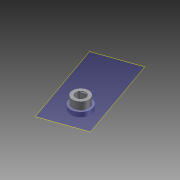
# Autodesk Inventor part: BlankLargeGearMotorInput
Saved by Autodesk Inventor 2012 (Build 160160000, 160)
## iProperties
Created: 2011-10-22
Part Number: BlankLargeGearMotorInput
Material: Default
Document SubType Name: Modeling
Designer: KuttaA
Density: 1 g/cm^3
Mass: 1.83252 g
Surface Area: 19.0134 cm^2
Volume: 1.83252 cm^3
Author: KuttaA
Autodesk Inventor part; units mm, degrees
ref_plane "YZ Plane" through (0, 0, 0) normal (1, 0, 0) x (0, 1, 0)
ref_plane "XZ Plane" through (0, 0, 0) normal (0, 1, 0) x (-1, 0, 0)
ref_plane "XY Plane" through (0, 0, 0) normal (0, 0, 1) x (1, 0, 0)
ref_plane "Work Plane1" through (-3.2804, 8.4734, 7) normal (0, 0, -1) x (0.3299562, -0.9439962, 0)
sketch "Sketch5" plane through (-3.2804, 8.4734, 7) normal (0, 0, -1) x (0.3299562, -0.9439962, 0)
  circle A0 centre (9.0812, -0.3009) radius 5.6 projected
  circle A1 centre (9.0812, -0.3009) radius 6.6
  point P0 (9.0812, -0.3009)
  dimension "d13" = 1
  constraints: 1 centre point, 1 coincident
  measures "d13" radial gap between concentric circles of A1 A0
extrude "Extrusion4" add sketch "Sketch5" along normal blind 3
sketch "Sketch6" plane through (0, 0, 7) normal (0, 0, 1) x (1, 0, 0)
  circle A0 centre (0, 0) radius 6.6 projected
  circle A1 centre (0, 0) radius 5.6 projected
  point P0 (0, 0)
extrude "Extrusion5" cut sketch "Sketch6" against normal blind 0.3
sketch "Sketch11" plane through (-3.2804, 8.4734, 7) normal (0, 0, -1) x (0.3299562, -0.9439962, 0)
  circle A0 centre (9.0812, -0.3009) radius 6.6
  circle A1 centre (9.0812, -0.3009) radius 3.3
  line L0 (6.3698, -2.1819) -> (6.3698, 1.5801)
  dimension "d26" = 13.2
  dimension "d27" = 6.6
  dimension "d28" = 3.762
  constraints: 2 centre point, 2 coincident, 2 end point, 2 point on circle, 1 vertical
  measures "d26" diameter of A0
  measures "d27" diameter of A1
  measures "d28" distance of L0.start L0.end
extrude "Extrusion10" add sketch "Sketch11" along normal blind 2.7 contours A0 | L0 A1 picked at (6.2456, 0.0906)
sketch "Sketch13" plane through (-3.2804, 8.4734, 7) normal (0, 0, -1) x (0.3299562, -0.9439962, 0)
  circle A0 centre (9.0812, -0.3009) radius 5.3
  arc A1 (6.3703, -2.1826) -> (6.3703, 1.5809) centre (9.0812, -0.3009) ccw projected
  line L0 (6.3703, 1.5809) -> (6.3703, -2.1826) projected
  dimension "d33" = 10.6
  constraints: 1 centre point, 1 coincident
  measures "d33" diameter of A0
extrude "Extrusion12" add sketch "Sketch13" against normal blind 5
sketch "Sketch14" plane through (0, 0, 4) normal (0, 0, -1) x (-1, 0, 0)
  line L0 (-0.881, 3.1802) -> (2.6703, 1.9389) projected
  arc A0 (-0.881, 3.1802) -> (2.6703, 1.9389) centre (0, 0) ccw projected
  circle A1 centre (0, 0) radius 5.6 projected
  point P0 (0, 0)
extrude "Extrusion13" add sketch "Sketch14" against normal up to surface (0.3 mm away)
sketch "Sketch15" plane through (0, 0, 12) normal (0, 0, 1) x (1, 0, 0)
  arc A0 (-2.6708, 1.9382) -> (0.8818, 3.18) centre (0, 0) ccw projected
  circle A1 centre (0, 0) radius 3.3
  point P0 (0, 0)
  constraints: 1 coincident, 3 other
extrude "Extrusion14" cut sketch "Sketch15" against normal blind 0.5
body "Solid1"
